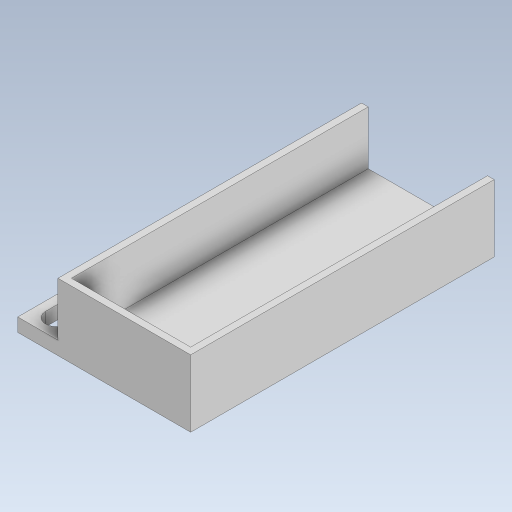
# Autodesk Inventor part: Mounting Relay
Saved by Autodesk Inventor 2023.5 (Build 275446000, 446)
## iProperties
Created: 2025-10-17
Part Number: Mounting Relay
Material: Generic
Document SubType Name: Modeling
Designer: Guntur
Density: 1 g/cm^3
Appearance: Default
Author: Guntur
Autodesk Inventor part; units mm, degrees
ref_plane "YZ Plane" through (0, 0, 0) normal (1, 0, 0) x (0, 1, 0)
ref_plane "XZ Plane" through (0, 0, 0) normal (0, 1, 0) x (-1, 0, 0)
ref_plane "XY Plane" through (0, 0, 0) normal (0, 0, 1) x (1, 0, 0)
sketch "Sketch1" plane through (0, 0, 0) normal (0, 1, 0) x (-1, 0, 0)
  line L0 (8.9, 21.65) -> (-8.9, 21.65)
  line L1 (-8.9, 21.65) -> (-8.9, -21.65)
  line L2 (-8.9, -21.65) -> (8.9, -21.65)
  line L3 (8.9, -21.65) -> (8.9, 21.65)
  line L4 (8.9, 21.65) -> (-8.9, -21.65) construction
  line L5 (-8.9, 21.65) -> (8.9, -21.65) construction
  line L6 (9.9, 22.65) -> (-9.9, 22.65)
  line L7 (-9.9, 22.65) -> (-9.9, -22.65)
  line L8 (-9.9, -22.65) -> (9.9, -22.65)
  line L9 (9.9, -22.65) -> (9.9, 22.65)
  line L10 (9.9, 22.65) -> (-9.9, -22.65) construction
  line L11 (-9.9, 22.65) -> (9.9, -22.65) construction
  line L12 (9.9, 22.65) -> (15.9, 22.65)
  line L13 (15.9, 22.65) -> (15.9, -22.65)
  line L14 (15.9, -22.65) -> (9.9, -22.65)
  line L15 (9.9, -22.65) -> (9.9, 22.65)
  line L16 (8.9, -21.65) -> (8.9, -22.65)
  line L17 (-8.9, -21.65) -> (-8.9, -22.65)
  line L18 (12.9, 19.85) -> (12.9, -20.15) construction
  line L19 (11.25, 19.85) -> (11.25, -20.15)
  line L20 (14.55, -20.15) -> (14.55, 19.85)
  arc A0 (14.55, 19.85) -> (11.25, 19.85) centre (12.9, 19.85) ccw
  arc A1 (11.25, -20.15) -> (14.55, -20.15) centre (12.9, -20.15) ccw
  point P0 (0, 0)
  point P1 (12.9, -0.15)
  point P2 (12.9, -22.65)
  dimension "d0" = 17.8
  dimension "d1" = 43.3
  dimension "d2" = 19.8
  dimension "d3" = 45.3
  dimension "d4" = 6
  dimension "d5" = 3.3
  dimension "d6" = 40
  dimension "d7" = 2.5
  constraints: 44 end point, 7 parallel, 6 midpoint, 6 perpendicular, 4 point on circle, 4 tangent, 3 horizontal, 2 centre point, 2 point on line
  measures "d0" distance of L2.end L1.end
  measures "d1" distance of L1.end L0.end
  measures "d2" distance of L8.end L7.end
  measures "d3" distance of L7.end L6.end
  measures "d4" distance of L13.end L14.end
  measures "d5" diameter of A1
  measures "d6" distance of L18.start L18.end
  measures "d7" distance of point (12.9, -22.65) L18.end
extrude "Extrusion1" add sketch "Sketch1" along normal blind 2 contours L3 L2 L1 L0 | L16 L8 L17 L2 | L9 L12 L13 L14
extrude "Extrusion2" add sketch "Sketch1" along normal blind 10 contours L0 L1 L17 L8 L7 L6 L9 L16 L3
body "Solid1"
